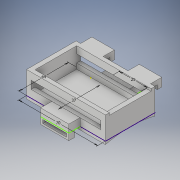
# Autodesk Inventor part: kotelon alaosa
Saved by Autodesk Inventor 2019 (Build 230136000, 136)
## iProperties
Created: 2018-07-23
Part Number: kotelon alaosa
Material: Generic
Document SubType Name: Modeling
Designer: OMISTAJA
Density: 1 g/cm^3
Appearance: Default
Author: OMISTAJA
## iProperties of the stored document kotelon alaosa_3DPrint.ipt
Created: 2018-07-24
Part Number: kotelon alaosa_3DPrint
Material: Generic
Document SubType Name: Modeling
Designer: OMISTAJA
Density: 1 g/cm^3
Appearance: Default
Author: OMISTAJA
Autodesk Inventor part; units mm, degrees
ref_plane "YZ Plane" through (0, 0, 0) normal (1, 0, 0) x (0, 1, 0)
ref_plane "XZ Plane" through (0, 0, 0) normal (0, 1, 0) x (-1, 0, 0)
ref_plane "XY Plane" through (0, 0, 0) normal (0, 0, 1) x (1, 0, 0)
sketch "Sketch1" plane through (0, 0, 0) normal (0, 1, 0) x (-1, 0, 0)
  line L0 (-31, -18.5) -> (31, -18.5)
  line L1 (31, -18.5) -> (31, 18.5)
  line L2 (31, 18.5) -> (-31, 18.5)
  line L3 (-31, 18.5) -> (-31, -18.5)
  line L4 (-31, -18.5) -> (31, 18.5) construction
  line L5 (31, -18.5) -> (-31, 18.5) construction
  line L6 (-35, -22) -> (35, -22)
  line L7 (35, -22) -> (35, 22)
  line L8 (35, 22) -> (-35, 22)
  line L9 (-35, 22) -> (-35, -22)
  line L10 (-35, -22) -> (35, 22) construction
  line L11 (35, -22) -> (-35, 22) construction
  line L12 (12.5, -32) -> (-12.5, -32)
  line L13 (0, -22) -> (12.5, -32) construction
  line L14 (0, -22) -> (-12.5, -32) construction
  line L15 (-12.5, 32) -> (12.5, 32)
  line L16 (12.5, 32) -> (12.5, 22)
  line L17 (-12.5, 22) -> (-12.5, 32)
  line L18 (-12.5, 32) -> (0, 22) construction
  line L19 (12.5, 32) -> (0, 22) construction
  line L20 (12.5, -22) -> (12.5, -32)
  line L21 (-12.5, -32) -> (-12.5, -22)
  line L22 (-12.5, -27) -> (12.5, -27)
  line L23 (-12.5, 27) -> (12.5, 27)
  line L24 (-35, -22) -> (-35, -18.5)
  line L25 (-35, 22) -> (-31, 22)
  line L26 (-35, 22) -> (-35, 18.5)
  point P0 (0, 0)
  dimension "d2" = 70
  dimension "d3" = 44
  dimension "d16" = 25
  dimension "d97" = 37
  constraints: 54 end point, 11 midpoint, 7 point on line, 6 parallel, 3 horizontal, 3 perpendicular, 2 collinear
  measures "d2" distance of L8.end L7.end
  measures "d3" distance of L7.end L6.end
  measures "d16" distance of L12.start L12.end
  measures "d97" distance between parallel lines of L2 L0
extrude "Extrusion2" add sketch "Sketch1" along normal blind 20 contours L9 L8 L7 L6
extrude "Extrusion3" add sketch "Sketch1" along normal blind 2 contours L3 L2 L1 L0
sketch "Sketch2" plane through (-35, 0, 22) normal (0, 0, 1) x (1, 0, 0)
  line L0 (66, 2) -> (66, 20) projected
  line L1 (4, 2) -> (4, 20) projected
  line L2 (66, 13.7796) -> (4, 13.7796)
  line L3 (4, 13.7796) -> (4, 6.7329)
  line L4 (4, 6.7329) -> (66, 6.7329)
  line L5 (66, 6.7329) -> (66, 13.7796)
  point P0 (35, 0)
  constraints: 8 end point, 2 parallel, 2 point on line, 1 horizontal, 1 perpendicular
extrude "Extrusion4" cut sketch "Sketch2" against normal blind 45
extrude "Extrusion5" add sketch "Sketch1" along normal blind 2 contours L6 L20 L22 L21 | L22 L20 L12 L21
extrude "Extrusion6" add sketch "Sketch1" along normal blind 2 contours L8 L17 L23 L16 | L23 L17 L15 L16
sketch "Sketch3" plane through (-12.5, 2, 32) normal (0, 0, 1) x (1, 0, 0)
  line L0 (2.5, -3.3793) -> (22.5, -3.3793)
  line L1 (22.5, -3.3793) -> (22.5, -4.9914)
  line L2 (22.5, -4.9914) -> (2.5, -4.9914)
  line L3 (2.5, -4.9914) -> (2.5, -3.3793)
  line L4 (25, -2) -> (25, 0) projected
  point P0 (12.5, -2)
  point P1 (25, -6)
  dimension "d28" = 20
  dimension "d29" = 2.5
  constraints: 8 end point, 2 parallel, 1 horizontal, 1 perpendicular
  measures "d28" distance of L1.end L2.end
  measures "d29" distance between parallel lines of L1 L4
extrude "Extrusion9" cut sketch "Sketch3" against normal blind 5
sketch "Sketch4" plane through (12.5, 2, -32) normal (0, 0, -1) x (-1, 0, 0)
  line L0 (2.5, -3.3796) -> (22.5, -3.3796)
  line L1 (22.5, -3.3796) -> (22.5, -4.9916)
  line L2 (22.5, -4.9916) -> (2.5, -4.9916)
  line L3 (2.5, -4.9916) -> (2.5, -3.3796)
  line L4 (25, -2) -> (25, 0) projected
  point P0 (12.5, -2)
  point P1 (25, -6)
  dimension "d32" = 20
  dimension "d34" = 2.5
  constraints: 8 end point, 2 parallel, 1 horizontal, 1 perpendicular
  measures "d32" distance of L1.end L2.end
  measures "d34" distance between parallel lines of L1 L4
extrude "Extrusion10" cut sketch "Sketch4" against normal blind 5
extrude "Extrusion11" add sketch "Sketch1" against normal blind 10 contours L9 L8 L7 L6
extrude "Extrusion12" add sketch "Sketch1" against normal blind 10 contours L3 L2 L1 L0
sketch "Sketch5" plane through (35, 20, 22) normal (1, 0, 0) x (0, 0, -1)
  line L0 (22, -20) -> (22, -110)
  circle A0 centre (22, -110) radius 90
  dimension "d42" = 90
  dimension "d43" = 180
  constraints: 2 end point, 1 centre point, 1 coincident, 1 vertical
  measures "d42" distance of L0.start L0.end
  measures "d43" diameter of A0
extrude "Extrusion13" cut sketch "Sketch5" against normal blind 70
sketch "Sketch6" plane through (35, 20, -22) normal (0, 0, -1) x (-1, 0, 0)
  point P0 (35, -20)
sketch "Sketch7" plane through (0, 20, 0) normal (0, 1, 0) x (1, 0, 0)
  line L0 (-31, 18.5) -> (31, 18.5) projected
  line L1 (31, 18.5) -> (35, 18.5)
  line L2 (35, -22) -> (35, 22) projected
  line L3 (31, 18.5) -> (31, -18.5) projected
  line L4 (31, -18.5) -> (36, -18.5)
  point P0 (0, 0)
  constraints: 4 end point, 2 horizontal, 1 point on line
sketch "Sketch8" plane through (31, 20, -18.5) normal (-1, 0, 0) x (0, 0, 1)
  line L0 (0, 0) -> (0, -2)
  line L1 (0, -2) -> (37, -2)
  line L2 (37, -6.2204) -> (37, 0) projected
  line L3 (37, -2) -> (37, 0)
  line L4 (37, -5.0018) -> (37, -7.0018)
  line L5 (40.5, 0) -> (-3.5, 0) projected
  line L6 (37, -7.0018) -> (2, -7.0018)
  line L7 (2, -7.0018) -> (2, -5.0018)
  point P0 (18.5, -20)
  dimension "d46" = 2
  dimension "d47" = 2
  constraints: 12 end point, 4 perpendicular, 2 point on line, 1 collinear, 1 vertical
  measures "d46" distance of L0.start L0.end
  measures "d47" distance of L4.start L4.end
sketch "Sketch14" plane through (0, 20, 0) normal (0, 1, 0) x (1, 0, 0)
  line L0 (31, 18.5) -> (31, 22) projected
  line L1 (31, 18.5) -> (35, 18.5)
  line L2 (35, -22) -> (35, 22) projected
  line L3 (31, 18.5) -> (31, -18.5) projected
  line L4 (31, -18.5) -> (35, -18.5)
  line L5 (35, -18.5) -> (35, 18.5)
  line L6 (31, 18.5) -> (31, -18.5)
  line L7 (-31, 18.5) -> (31, 18.5) projected
  line L8 (31, -18.5) -> (-31, -18.5) projected
  line L9 (31, -18.5) -> (31, -14.9394)
  constraints: 10 end point, 2 horizontal, 2 point on line, 1 parallel, 1 perpendicular
extrude "Extrusion18" cut sketch "Sketch14" against normal blind 2
sketch "Sketch21" plane through (35, -2.7303, -22) normal (0, 0, -1) x (-1, 0, 0)
  line L0 (66, 15.2303) -> (66, 19.6201)
  line L1 (66, 16.5099) -> (66, 22.7303) projected
  line L2 (66, 22.7303) -> (46, 22.7303)
  line L3 (46, 22.7303) -> (46, 15.2303)
  line L4 (46, 15.2303) -> (66, 15.2303)
  line L5 (66, 22.7303) -> (66, 15.2303)
  point P0 (35, 2.7303)
  dimension "d84" = 7.5
  dimension "d91" = 20
  constraints: 10 end point, 1 collinear, 1 midpoint, 1 perpendicular, 1 point on line, 1 vertical
  measures "d84" distance of L2.end L3.end
  measures "d91" distance between parallel lines of L3 L0
sketch "Sketch25" plane through (31, 6.7329, -22) normal (0, 0, -1) x (-1, 0, 0)
  line L0 (0, 7.0467) -> (62, 7.0467) projected
  line L1 (0, 7.0467) -> (0, 13.2671)
  line L2 (66, 13.2671) -> (-4, 13.2671) projected
  line L3 (0, 13.2671) -> (20, 13.2671)
  line L4 (20, 13.2671) -> (20, 5.7671)
  line L5 (20, 5.7671) -> (0, 5.7671)
  line L6 (0, 5.7671) -> (0, 13.2671)
  point P0 (31, -6.7329)
  dimension "d98" = 20
  dimension "d99" = 7.5
  constraints: 10 end point, 2 perpendicular, 2 point on line, 1 collinear, 1 vertical
  measures "d98" distance of L1.end L3.end
  measures "d99" distance of L3.end L4.end
extrude "Extrusion29" add sketch "Sketch1" against normal blind 6 contours L22 L20 L12 L21
extrude "Extrusion30" add sketch "Sketch1" against normal blind 6 contours L23 L17 L15 L16
sketch "Sketch28" plane through (12.5, 2, -32) normal (0, 0, -1) x (-1, 0, 0)
  line L0 (2, -3.2303) -> (23, -3.2303)
  line L1 (23, -3.2303) -> (23, -6.2303)
  line L2 (23, -6.2303) -> (2, -6.2303)
  line L3 (2, -6.2303) -> (2, -3.2303)
  line L4 (-22.5, -4.7303) -> (47.5, -4.7303) projected
  line L5 (2, -3.2303) -> (23, -6.2303) construction
  line L6 (23, -3.2303) -> (2, -6.2303) construction
  point P0 (12.5, -2)
  point P1 (12.5, -4.7303)
  dimension "d111" = 21
  dimension "d112" = 3
  constraints: 12 end point, 3 midpoint, 2 parallel, 1 horizontal, 1 perpendicular
  measures "d111" distance of L1.end L2.end
  measures "d112" distance of L0.end L1.end
extrude "Extrusion31" cut sketch "Sketch28" against normal blind 6
sketch "Sketch29" plane through (-12.5, 2, 32) normal (0, 0, 1) x (1, 0, 0)
  line L0 (2, -3.2303) -> (23, -3.2303) projected
  line L1 (2, -6.2303) -> (23, -6.2303)
  line L2 (23, -6.2303) -> (23, -3.2303)
  line L3 (23, -3.2303) -> (2, -3.2303)
  line L4 (2, -3.2303) -> (2, -6.2303)
  line L5 (47.5, -4.7303) -> (-22.5, -4.7303) projected
  line L6 (2, -6.2303) -> (23, -3.2303) construction
  line L7 (23, -6.2303) -> (2, -3.2303) construction
  point P0 (12.5, -2)
  point P1 (12.5, -4.7303)
  dimension "d115" = 21
  constraints: 12 end point, 3 midpoint, 2 parallel, 1 horizontal, 1 perpendicular
  measures "d115" distance of L3.end L0.end
extrude "Extrusion32" cut sketch "Sketch29" against normal blind 6
sketch "Sketch30" plane through (-12.5, 0, -22) normal (-1, 0, 0) x (0, 0, 1)
  point P0 (22, 0)
extrude "Extrusion33" cut sketch "Sketch1" along normal blind 6.75 contours L8 L17 L23 L16 | L23 L17 L15 L16
extrude "Extrusion34" add sketch "Sketch1" along normal blind 6.75 contours L23 L17 L15 L16
extrude "Extrusion35" add sketch "Sketch1" along normal blind 6.75 contours L8 L17 L23 L16
extrude "Extrusion36" cut sketch "Sketch1" along normal blind 6.75 contours L6 L20 L22 L21
extrude "Extrusion37" add sketch "Sketch1" along normal blind 6.75 contours L6 L20 L22 L21 | L22 L20 L12 L21
extrude "Extrusion38" add sketch "Sketch25" along normal blind 10
extrude "Extrusion39" add sketch "Sketch21" along normal blind 10
sketch "Sketch32" plane through (-31, 13.7796, -22) normal (-1, 0, 0) x (0, 0, 1)
  line L0 (-10, 6.2204) -> (-10, -1.2796) projected
  line L1 (-6, 2.4704) -> (0, 2.4704)
  line L2 (0, -16.5099) -> (0, 6.2204) projected
  line L3 (-6, 2.4704) -> (-6, -1.2796)
  line L4 (0, -1.2796) -> (-10, -1.2796) projected
  line L5 (-6, -1.2796) -> (0, -1.2796)
  line L6 (0, 2.4704) -> (0, -1.2796)
  point P0 (22, -13.7796)
  constraints: 8 end point, 2 collinear, 2 point on line, 1 horizontal
extrude "Extrusion40" cut sketch "Sketch32" against normal blind 20
sketch "Sketch33" plane through (31, 13.7796, -22) normal (1, 0, 0) x (0, 0, -1)
  line L0 (10, -1.2796) -> (10, 6.2204) projected
  line L1 (0, 2.4704) -> (6, 2.4704) projected
  line L2 (6, 2.4704) -> (6, -1.2796) projected
  line L3 (6, 2.4704) -> (6, -1.2796)
  line L4 (6, -1.2796) -> (6, 2.4704)
  line L5 (6, -1.2796) -> (0, -1.2796)
  line L6 (0, -1.2796) -> (0, 2.4704)
  line L7 (6, 2.4704) -> (0, 2.4704)
  point P0 (-22, -13.7796)
  constraints: 10 end point, 2 collinear, 1 horizontal, 1 perpendicular
extrude "Extrusion41" cut sketch "Sketch33" against normal blind 20
sketch "Sketch34" plane through (0, 20, 0) normal (0, 1, 0) x (1, 0, 0)
  point P0 (0, 0)
body "Solid2"
